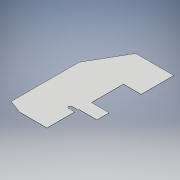
# Autodesk Inventor part: Gearbox-Side Cover Part 1
Saved by Autodesk Inventor 2018 (Build 220112000, 112)
## iProperties
Created: 2018-08-07
Part Number: Gearbox-Side Cover Part 1
Material: Generic
Document SubType Name: Modeling
Designer: P301319
Density: 1 g/cm^3
Appearance: Default
Author: P301319
Autodesk Inventor part; units mm, degrees
ref_plane "YZ Plane" through (0, 0, 0) normal (1, 0, 0) x (0, 1, 0)
ref_plane "XZ Plane" through (0, 0, 0) normal (0, 1, 0) x (-1, 0, 0)
ref_plane "XY Plane" through (0, 0, 0) normal (0, 0, 1) x (1, 0, 0)
sketch "Sketch1" plane through (0, 0, 0) normal (0, 0, 1) x (1, 0, 0)
  line L0 (0, 0) -> (200, 0)
  line L1 (0, 0) -> (-100, 36.397)
  line L2 (0, 0) -> (236.9147, 0) construction
  line L3 (-100, 536.397) -> (-100, 36.397)
  line L4 (-100, 536.397) -> (52.1912, 800)
  line L5 (-100, 536.397) -> (462.0527, 536.397) construction
  line L6 (52.1912, 800) -> (332.1912, 800)
  line L7 (332.1912, 800) -> (332.1912, 560)
  line L8 (332.1912, 560) -> (202.1912, 560)
  line L9 (202.1912, 560) -> (202.1912, 325)
  line L10 (202.1912, 325) -> (332.1912, 325)
  line L11 (200, 235) -> (332.1912, 235)
  line L12 (332.1912, 325) -> (332.1912, 235)
  line L13 (155, 203.5) -> (200, 203.5)
  line L14 (155, 228.5) -> (200, 228.5)
  arc A0 (155, 228.5) -> (155, 203.5) centre (155, 216) ccw
  line L15 (200, 0) -> (200, 203.5)
  line L16 (200, 228.5) -> (200, 235)
  dimension "d0" = 200
  dimension "d1" = 160
  dimension "d2" = 500
  dimension "d3" = 100
  dimension "d4" = 60
  dimension "d5" = 280
  dimension "d6" = 800
  dimension "d7" = 240
  dimension "d8" = 130
  dimension "d9" = 235
  dimension "d10" = 130
  dimension "d11" = 235
  dimension "d14" = 25
  dimension "d16" = 216
  dimension "d18" = 45
  constraints: 36 end point, 7 horizontal, 5 perpendicular, 3 vertical, 2 point on circle, 2 tangent, 1 centre point, 1 parallel, 1 vertical alignment
  measures "d0" distance of L0.start L0.end
  measures "d1" angle of L2 L1
  measures "d2" distance of L1.end L3.start
  measures "d3" distance from line of L0.start L3
  measures "d4" angle of L5 L4
  measures "d5" distance of L4.end L6.end
  measures "d6" distance between parallel lines of L0 L6
  measures "d7" distance of L6.end L7.end
  measures "d8" distance of L7.end L8.end
  measures "d9" distance of L8.end L9.end
  measures "d10" distance of L9.end L10.end
  measures "d11" distance of L0.end L11.start
  measures "d14" distance between parallel lines of L13 L14
  measures "d16" vertical distance of L0.start A0.centre
  measures "d18" distance of L13.start L13.end
extrude "Extrusion1" add sketch "Sketch1" along normal blind 1.6
equation "\"d10\" = d8"
body "Solid1"
